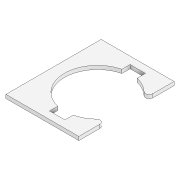
# Autodesk Inventor part: Adapt_Roue_libre
Saved by Autodesk Inventor 2022 (Build 260153000, 153)
## iProperties
Created: 2021-03-03
Part Number: Adapt_Roue_libre
Material: Générique
Document SubType Name: Modeling
Designer: utilisateur
Density: 1 g/cm^3
Appearance: Par défaut(1)
Author: utilisateur
Autodesk Inventor part; units mm, degrees
ref_plane "YZ Plane" through (0, 0, 0) normal (1, 0, 0) x (0, 1, 0)
ref_plane "XZ Plane" through (0, 0, 0) normal (0, 1, 0) x (-1, 0, 0)
ref_plane "XY Plane" through (0, 0, 0) normal (0, 0, 1) x (1, 0, 0)
sketch "Esquisse1" plane through (0, 0, 0) normal (1, 0, 0) x (0, 1, 0)
  line L0 (0.5, 12) -> (-0.5, 12)
  line L1 (-0.5, 12) -> (-0.5, -12)
  line L2 (-0.5, -12) -> (0.5, -12)
  line L3 (0.5, -12) -> (0.5, 12)
  line L4 (0.5, 12) -> (-0.5, -12) construction
  line L5 (-0.5, 12) -> (0.5, -12) construction
  line L6 (0.5, -12) -> (-4.7, -12)
  line L7 (-4.7, -12) -> (-4.7, -13)
  line L8 (-4.7, -13) -> (0.5, -13)
  line L9 (0.5, -13) -> (0.5, -12)
  line L10 (0.5, 12) -> (-4.7, 12)
  line L11 (-4.7, 12) -> (-4.7, 13)
  line L12 (-4.7, 13) -> (0.5, 13)
  line L13 (0.5, 13) -> (0.5, 12)
  line L14 (-4.7, -13) -> (-3.7, -13)
  line L15 (-3.7, -13) -> (-3.7, -21)
  line L16 (-3.7, -21) -> (-4.7, -21)
  line L17 (-4.7, -21) -> (-4.7, -13)
  line L18 (-4.7, 13) -> (-3.7, 13)
  line L19 (-3.7, 13) -> (-3.7, 21)
  line L20 (-3.7, 21) -> (-4.7, 21)
  line L21 (-4.7, 21) -> (-4.7, 13)
  point P0 (0, 0)
  dimension "d0" = 24
  dimension "d1" = 1
  dimension "d2" = 8
  dimension "d3" = 4.2
  constraints: 44 end point, 10 parallel, 6 equal length, 5 horizontal, 5 perpendicular, 2 midpoint, 1 point on line
  measures "d0" distance between parallel lines of L6 L10
  measures "d1" distance of L0.start L0.end
  measures "d2" distance of L14.end L15.end
  measures "d3" distance between parallel lines of L11 L1
extrude "Extrusion1" add sketch "Esquisse1" along normal mid plane 15.8
sketch "Esquisse2" plane through (-7.9, -0.5, -12) normal (0, -1, 0) x (1, 0, 0)
  circle A0 centre (7.9, 19.9) radius 2.1
  line L0 (7.9, 19.9) -> (7.9, 12) construction
  line L1 (7.9, 12) -> (7.9, 4.1) construction
  line L2 (10, 19.9) -> (10, 24)
  line L3 (0, 24) -> (15.8, 24) projected
  line L4 (5.8, 24) -> (5.8, 19.9)
  line L5 (10, 19.9) -> (5.8, 19.9) construction
  dimension "d6" = 15.8
  dimension "d7" = 4.2
  constraints: 10 end point, 3 point on line, 3 vertical, 2 point on circle, 1 centre point, 1 collinear, 1 horizontal, 1 tangent
  measures "d6" distance of L1.end L0.start
  measures "d7" diameter of A0
extrude "Extrusion2" cut sketch "Esquisse2" against normal through all
sketch "Esquisse3" plane through (-7.9, -3.7, 21) normal (0, 1, 0) x (1, 0, 0)
  circle A0 centre (7.9, 4) radius 1.6
  line L0 (0, 0) -> (15.8, 0) construction
  line L1 (7.9, 0) -> (7.9, 4) construction
  line L2 (7.9, 4) -> (7.9, 8) construction
  line L3 (0, 8) -> (15.8, 8) construction
  point P0 (7.9, 21)
  dimension "d10" = 3.2
  constraints: 4 end point, 2 midpoint, 2 vertical, 1 centre point, 1 collinear
  measures "d10" diameter of A0
extrude "Extrusion3" cut sketch "Esquisse3" against normal through all
mirror "Symétrie2" about plane through (0, 0, 0) normal (0, 0, 1) of "Extrusion2", "Extrusion3"
sketch "Sketch4" plane through (7.9, 0, 0) normal (1, 0, 0) x (0, 0, -1)
  line L0 (13, 0.5) -> (-13, 0.5) projected
  line L1 (-13, 0.5) -> (-13, -3.7) projected
  line L2 (-13, -3.7) -> (-21, -3.7) projected
  line L3 (-21, -3.7) -> (-21, -4.7) projected
  line L4 (-21, -4.7) -> (-12, -4.7) projected
  line L5 (-12, -4.7) -> (-12, -0.5) projected
  line L6 (-12, -0.5) -> (12, -0.5) projected
  line L7 (12, -0.5) -> (12, -4.7) projected
  line L8 (12, -4.7) -> (21, -4.7) projected
  line L9 (21, -4.7) -> (21, -3.7) projected
  line L10 (21, -3.7) -> (13, -3.7) projected
  line L11 (13, -3.7) -> (13, 0.5) projected
  line L12 (-12, -0.5) -> (-13, -0.5)
  line L13 (12, -0.5) -> (13, -0.5)
  point P0 (0, 0)
  constraints: 4 end point, 2 perpendicular, 2 point on line
extrude "Extrusion4" cut sketch "Sketch4" against normal through all contours L11 L10 L9 L8 L7 L13 | L12 L5 L4 L3 L2 L1
sketch "Sketch5" plane through (-7.9, 0.5, 13) normal (0, 1, 0) x (1, 0, 0)
  line L0 (-4.1, 0) -> (19.9, 0)
  line L1 (19.9, 0) -> (19.9, 26)
  line L2 (19.9, 26) -> (-4.1, 26)
  line L3 (-4.1, 26) -> (-4.1, 0)
  line L4 (-4.1, 0) -> (19.9, 26) construction
  line L5 (19.9, 0) -> (-4.1, 26) construction
  arc A0 (5.8, 20.9) -> (10, 20.9) centre (7.9, 20.9) ccw projected
  line L6 (5.8, 20.9) -> (5.8, 25) projected
  line L7 (5.8, 25) -> (10, 25) projected
  line L8 (10, 25) -> (10, 20.9) projected
  line L9 (10, 1) -> (5.8, 1) projected
  line L10 (5.8, 1) -> (5.8, 5.1) projected
  arc A1 (10, 5.1) -> (5.8, 5.1) centre (7.9, 5.1) ccw projected
  line L11 (10, 5.1) -> (10, 1) projected
  line L12 (0, 0) -> (15.8, 0) projected
  line L13 (15.8, 26) -> (15.8, 0) projected
  line L14 (15.8, 26) -> (0, 26) projected
  line L15 (0, 0) -> (0, 26) projected
  point P0 (7.9, 13)
  dimension "d16" = 24
  dimension "d22" = 26
  constraints: 12 end point, 2 midpoint, 2 parallel, 1 horizontal, 1 perpendicular
  measures "d16" distance of L1.end L2.end
  measures "d22" distance of L0.end L1.end
extrude "Extrusion5" add sketch "Sketch5" against normal up to surface (1 mm away) contours L3 L2 L15 L0 | L13 L2 L1 L0
sketch "Sketch7" plane through (-12, 0.5, -13) normal (0, 1, 0) x (1, 0, 0)
  circle A0 centre (12, -13) radius 9
  dimension "d23" = 18
  constraints: 1 centre point, 1 coincident
  measures "d23" diameter of A0
extrude "Extrusion7" cut sketch "Sketch7" against normal through all
sketch "Sketch8" plane through (12, 0.5, 13) normal (0, 1, 0) x (1, 0, 0)
  line L0 (-24, 0) -> (0, 0) projected
  line L1 (0, 0) -> (0, 26) projected
  line L2 (0, 26) -> (-24, 26) projected
  line L3 (-24, 26) -> (-24, 0) projected
  arc A0 (-9.9, 4.2484) -> (-9.9, 21.7516) centre (-12, 13) ccw projected
  line L4 (-9.9, 4.2484) -> (-9.9, 1) projected
  line L5 (-9.9, 1) -> (-14.1, 1) projected
  line L6 (-14.1, 1) -> (-14.1, 4.2484) projected
  arc A1 (-14.1, 21.7516) -> (-14.1, 4.2484) centre (-12, 13) ccw projected
  line L7 (-14.1, 21.7516) -> (-14.1, 25) projected
  line L8 (-14.1, 25) -> (-9.9, 25) projected
  line L9 (-9.9, 25) -> (-9.9, 21.7516) projected
  line L10 (-14.1, 2) -> (-9.9, 2)
  line L11 (-14.1, 24) -> (-9.9, 24)
  line L12 (-12, 2) -> (-12, 1) construction
  line L13 (-12, 24) -> (-12, 25) construction
  point P0 (-14.1, 24)
  dimension "d27" = 1
  constraints: 8 end point, 4 midpoint, 3 point on line, 1 collinear, 1 horizontal, 1 perpendicular, 1 vertical
  measures "d27" distance between parallel lines of L5 L10
extrude "Extrusion9" add sketch "Sketch8" against normal up to surface (1 mm away) contours L4 L5 L6 L10 | L11 L7 L8 L9
sketch "Sketch9" plane through (12, 0.5, 13) normal (0, 1, 0) x (1, 0, 0)
  line L0 (-24, 0) -> (0, 0) projected
  line L1 (0, 0) -> (0, 26) projected
  line L2 (0, 26) -> (-24, 26) projected
  line L3 (-24, 26) -> (-24, 0) projected
  arc A0 (-9.9, 4.2484) -> (-9.9, 21.7516) centre (-12, 13) ccw projected
  line L4 (-9.9, 4.2484) -> (-9.9, 2) projected
  line L5 (-9.9, 2) -> (-14.1, 2) projected
  line L6 (-14.1, 2) -> (-14.1, 4.2484) projected
  arc A1 (-14.1, 21.7516) -> (-14.1, 4.2484) centre (-12, 13) ccw projected
  line L7 (-14.1, 21.7516) -> (-14.1, 24) projected
  line L8 (-14.1, 24) -> (-9.9, 24) projected
  line L9 (-9.9, 24) -> (-9.9, 21.7516) projected
  line L10 (0, 26) -> (-4.1, 26)
  line L11 (-4.1, 26) -> (-4.1, 0)
  line L12 (-4.1, 0) -> (0, 0)
  line L13 (0, 0) -> (0, 26)
  point P0 (-4.1, 8.6884)
  point P1 (-4.1, 17.3116)
  dimension "d32" = 4.1
  constraints: 8 end point, 2 parallel, 1 horizontal, 1 perpendicular, 1 point on line
  measures "d32" distance of L1.end L10.end
extrude "Extrusion10" cut sketch "Sketch9" against normal through all contours L11 A0 L2 L1 L0
fillet "Fillet3" radius 1 2 edges at (7.9, 0, 4.3116) (7.9, 0, -4.3116)
